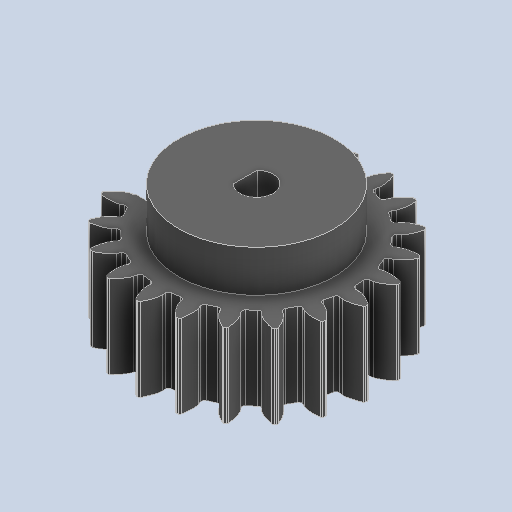
# Autodesk Inventor part: screw_gear_under
Saved by Autodesk Inventor 2024.1 (Build 281209000, 209)
## iProperties
Created: 2025-01-10
Part Number: screw_gear_under
Material: 一般
Document SubType Name: Modeling
Designer: hibik
Density: 1 g/cm^3
Appearance: 既定
Author: hibik
Autodesk Inventor part; units mm, degrees
ref_plane "XZ Plane" through (0, 0, 0) normal (0, 1, 0) x (-1, 0, 0)
sketch "スケッチ1" plane through (0, 0, 0) normal (0, 1, 0) x (-1, 0, 0)
  circle A0 centre (0, 0) radius 10.5 construction
  circle A1 centre (0, 0) radius 9.8668 construction
  line L0 (0, 0) -> (0.7373, -9.8392)
  line L1 (0, -18.6437) -> (0, 15.3573) projected
  dimension "d1" = 19.7336
  dimension "d0" = 21
  dimension "d4" = 4.286
  constraints: 3 coincident, 2 end point, 1 centre point, 7 other
  measures "d0" diameter of A0
  measures "d4" angle of L1 L0
sketch "スケッチ2" plane through (0, 0, 0) normal (0, 1, 0) x (-1, 0, 0)
  circle A0 centre (0, 0) radius 11.5
  dimension "d5" = 23
  constraints: 1 centre point, 1 coincident
  measures "d5" diameter of A0
extrude "押し出し1" add sketch "スケッチ2" along normal blind 8
sketch "スケッチ3" plane through (0, 8, 0) normal (0, 1, 0) x (1, 0, 0)
  line L0 (0, 0) -> (-0.7373, 9.8392) projected
  spline S0 degree 3 poles (-0.7373, 9.8392) (-0.7373, 9.8392) (-0.7943, 10.4208) (-1.4495, 11.2846) (-1.9355, 11.9253) (-2.7502, 12.7069) (-3.9821, 13.3735) knots 0 0 0 0 0.574125 0.574125 0.574125 1 1 1 1 projected
  circle A0 centre (0, 0) radius 11.5 projected
  circle A1 centre (0, 0) radius 9.25
  line L1 (0, 18.8437) -> (0, -16.5573) projected
  point P0 (0, 9.25)
  point P1 (0, 11.5)
  point P2 (-1.5369, 11.3968)
  point P3 (-0.6913, 9.2241)
  dimension "d10" = 18.5
  constraints: 3 coincident, 1 centre point
  measures "d10" diameter of A1
extrude "押し出し2" cut sketch "スケッチ3" against normal through all contours L0 S0 A0 L1 A1 picked at (-0.2602, 10.2625)
fillet "フィレット1" radius 0.3 1 edges at (-0.6913, 4, -9.2241)
chamfer "面取り1" distance 0.1 angle 45 1 edges at (-1.5369, 4, -11.3968)
mirror "ミラー1" about plane through (0, 8, -11.5) normal (-1, 0, 0) of "押し出し2", "フィレット1", "面取り1"
pattern_circular "円形状パターン1" count 21 over 360 about axis through (0, -10, 0) along (0, 1, 0) of "押し出し2", "フィレット1", "面取り1", "ミラー1"
sketch "スケッチ4" plane through (0, 8, 0) normal (0, 1, 0) x (1, 0, 0)
  circle A0 centre (0, 0) radius 7.5
  dimension "d20" = 15
  constraints: 1 centre point, 1 coincident
  measures "d20" diameter of A0
extrude "押し出し3" add sketch "スケッチ4" along normal blind 4
sketch "スケッチ5" plane through (0, 12, 0) normal (0, 1, 0) x (1, 0, 0)
  circle A0 centre (0, 0) radius 1.6
  dimension "d23" = 3.2
  constraints: 1 centre point, 1 coincident
  measures "d23" diameter of A0
extrude "押し出し4" cut sketch "スケッチ5" against normal through all
sketch "スケッチ6" plane through (0, 0, 0) normal (0, -1, 0) x (1, 0, 0)
  circle A0 centre (0, 0) radius 5
  dimension "d26" = 10
  constraints: 1 centre point, 1 coincident
  measures "d26" diameter of A0
extrude "押し出し5" cut sketch "スケッチ6" against normal blind 3
sketch "スケッチ7" plane through (0, 0, 0) normal (1, 0, 0) x (0, 1, 0)
  line L0 (12, -7.5) -> (12, 7.5) projected
  line L1 (3, -5) -> (3, 5) projected
  circle A0 centre (7.5, 0) radius 0.85
  line L2 (12, 0) -> (3, 0) construction
  point P0 (0, 0)
  dimension "d29" = 1.7
  constraints: 3 midpoint, 2 end point, 1 centre point, 1 coincident, 1 horizontal alignment
  measures "d29" diameter of A0
extrude "押し出し6" cut sketch "スケッチ7" against normal through all
ref_plane "作業平面1" through (-3, 0, 0) normal (1, 0, 0) x (0, 1, 0)
sketch "スケッチ8" plane through (-3, 0, 0) normal (1, 0, 0) x (0, 1, 0)
  circle A0 centre (7.5, 0) radius 2.75
  line L0 (12, 1.6) -> (12, -1.6) projected
  line L1 (3, 1.6) -> (3, -1.6) projected
  line L2 (3, -5) -> (3, 5) projected
  line L3 (12, 0) -> (3, 0) construction
  line L4 (3, 1.6) -> (3, -1.6) projected
  point P0 (0, 0)
  point P1 (4.5, 0.85)
  point P2 (3, 2.3049)
  point P3 (3, -2.3049)
  dimension "d33" = 5.5
  constraints: 3 midpoint, 2 end point, 1 centre point, 1 coincident, 1 horizontal alignment, 1 vertical alignment, 7 other
  measures "d33" diameter of A0
extrude "押し出し7" cut sketch "スケッチ8" against normal through all
ref_plane "作業平面2" through (-1.1, 0, 0) normal (1, 0, 0) x (0, 1, 0)
sketch "スケッチ9" plane through (-1.1, 0, 0) normal (1, 0, 0) x (0, 1, 0)
  line L0 (12, -7.5) -> (12, 7.5) projected
  line L1 (3, -5) -> (3, 5) projected
  line L2 (3, -1.5) -> (12, -1.5)
  line L3 (12, -1.5) -> (12, 1.5)
  line L4 (12, 1.5) -> (3, 1.5)
  line L5 (3, 1.5) -> (3, -1.5)
  line L6 (3, 0) -> (12, 0)
  spline S0 degree 5 poles (8.35, 0) (8.35, 0.1675) (8.3085, 0.3349) (8.2273, 0.4797) (8.1235, 0.5973) (7.914, 0.7501) (7.8179, 0.7993) (7.7147, 0.8329) (7.6074, 0.85) (7.3927, 0.85) (7.2855, 0.8329) (7.1823, 0.7994) (7.0863, 0.7503) (6.9338, 0.6392) (6.8733, 0.5831) (6.8192, 0.5193) (6.7728, 0.4484) (6.7026, 0.3037) (6.6767, 0.2315) (6.6589, 0.1557) (6.65, 0.078) (6.65, -0.1675) (6.6915, -0.3349) (6.7727, -0.4797) (6.8765, -0.5973) (7.086, -0.7501) (7.1821, -0.7993) (7.2853, -0.8329) (7.3926, -0.85) (7.6073, -0.85) (7.7145, -0.8329) (7.8177, -0.7994) (7.9137, -0.7503) (8.0662, -0.6392) (8.1267, -0.5831) (8.1808, -0.5193) (8.2272, -0.4484) (8.2974, -0.3037) (8.3233, -0.2315) (8.3411, -0.1557) (8.35, -0.078) (8.35, 0) knots 0 0 0 0 0 0 0.146408 0.146408 0.146408 0.146408 0.250229 0.250229 0.250229 0.250229 0.353974 0.353974 0.353974 0.353974 0.432259 0.432259 0.432259 0.432259 0.500333 0.500333 0.500333 0.500333 0.646546 0.646546 0.646546 0.646546 0.750229 0.750229 0.750229 0.750229 0.853836 0.853836 0.853836 0.853836 0.932017 0.932017 0.932017 0.932017 1 1 1 1 1 1 projected
  line L7 (3, 1.6) -> (3, -1.6) projected
  line L8 (12, 1.6) -> (12, -1.6) projected
  point P0 (0, 0)
  point P1 (6, 2.3049)
  point P2 (6, -2.3049)
  point P3 (3, 2.3049)
  point P4 (3, -2.3049)
  dimension "d37" = 3
  constraints: 10 end point, 4 midpoint, 2 horizontal, 2 parallel, 1 perpendicular, 1 point on line, 4 other
  measures "d37" distance between parallel lines of L4 L2
extrude "押し出し8" add sketch "スケッチ9" against normal up to surface (1.9 mm away) contours L2 L1 L6 S0 L0 | L6 S0 L1 L4 L0
equation "\"module\" = 1"
